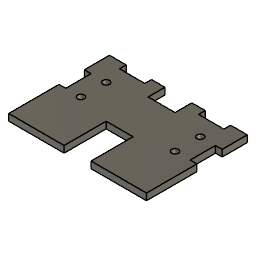
ultra Top (Autodesk Fusion 360 design; units mm, degrees)
part number: 2026-03-26-08-39-18-993
Autodesk Fusion 360 part; units mm, degrees
sketch "Sketch1" plane through (0, 0, 0) normal (0, 0, 1) x (1, 0, 0)
  circle A0 centre (27.5702, 32.2128) radius 2
  circle A1 centre (27.5702, 17.2128) radius 2
  circle A2 centre (83.5354, 17.2128) radius 2
  circle A3 centre (83.5354, 32.2128) radius 2
  line L0 (14.5612, 17.2128) -> (18.5612, 17.2128)
  line L1 (18.5612, 17.2128) -> (18.5612, 32.2128)
  line L2 (18.5612, 32.2128) -> (14.5612, 32.2128)
  line L3 (96.5612, 17.2128) -> (92.5612, 17.2128)
  line L4 (92.5612, 17.2128) -> (92.5612, 32.2128)
  line L5 (92.5612, 32.2128) -> (96.5612, 32.2128)
  line L6 (14.5612, 32.2128) -> (14.5612, 34.134)
  line L7 (14.5612, 34.134) -> (14.5612, 47.2128)
  line L8 (14.5612, 17.2128) -> (14.5612, -12.7872)
  line L9 (96.5612, -12.7872) -> (96.5612, 4.1678)
  line L10 (96.5612, 4.1678) -> (96.5612, 17.2128)
  line L11 (96.5612, 32.2128) -> (96.5612, 47.2128)
  line L12 (47.5702, 37.2128) -> (63.5354, 37.2128)
  line L13 (63.5354, 37.2128) -> (63.5354, 47.2128)
  line L14 (47.5702, 47.2128) -> (47.5702, 37.2128)
  line L15 (63.5354, 12.2128) -> (47.5702, 12.2128)
  line L16 (47.5702, 12.2128) -> (47.5702, -12.7872)
  line L17 (63.5354, -12.7872) -> (63.5354, 12.2128)
  line L18 (96.5612, -12.7872) -> (63.5354, -12.7872)
  line L19 (47.5702, -12.7872) -> (14.5612, -12.7872)
  line L20 (39.5612, 47.2128) -> (39.5612, 43.2128)
  line L21 (39.5612, 43.2128) -> (24.5612, 43.2128)
  line L22 (24.5612, 43.2128) -> (24.5612, 47.2128)
  line L23 (86.5612, 47.2128) -> (86.5612, 43.2128)
  line L24 (86.5612, 43.2128) -> (71.5444, 43.2128)
  line L25 (71.5444, 43.2128) -> (71.5444, 47.2128)
  line L26 (24.5612, 47.2128) -> (14.5612, 47.2128)
  line L27 (39.5612, 47.2128) -> (47.5702, 47.2128)
  line L28 (63.5354, 47.2128) -> (71.5444, 47.2128)
  line L29 (86.5612, 47.2128) -> (96.5612, 47.2128)
  dimension "d45" = 30
  dimension "d46" = 30
  constraint horizontal L0
  constraint vertical L1
  constraint horizontal L2
  constraint horizontal L3
  constraint vertical L4
  constraint horizontal L5
  constraint perpendicular L3 L10
  constraint horizontal L12
  constraint vertical L13
  constraint vertical L14
  constraint horizontal L15
  constraint vertical L16
  constraint vertical L17
  constraint perpendicular L8 L19
  constraint vertical L20
  constraint horizontal L21
  constraint vertical L22
  constraint vertical L23
  constraint horizontal L24
  constraint vertical L25
  constraint perpendicular L7 L26
  constraint perpendicular L25 L28
  constraint perpendicular L11 L29
  measures "d45" distance of L0.end L19
  measures "d46" distance of L3 L18
extrude "Extrude9" add sketch "Sketch1" along normal blind 4
